Autodesk Inventor part; units mm, degrees
(part 2 of 2)
sketch "Sketch11" plane through (0, 0, 0) normal (0, -1, 0) x (1, 0, 0)
  line L0 (-38.5, 57.5) -> (38.5, 57.5) construction
  line L1 (-38.5, 57.5) -> (-38.5, -57.5) construction
  line L2 (-32.0325, -46.9289) -> (-28.4969, -50.4645)
  line L3 (-28.4969, -50.4645) -> (-32.0325, -54)
  line L4 (-32.0325, -54) -> (-35.568, -50.4645)
  line L5 (-35.568, -50.4645) -> (-32.0325, -46.9289)
  line L6 (31.4645, 54) -> (35, 54) construction
  line L7 (-38.5, -54) -> (35, -54) construction
  line L8 (35, 54) -> (-38.5, 54)
  line L9 (-38.5, 54) -> (-38.5, -54) construction
  line L10 (-22.9615, -46.9289) -> (-19.4259, -50.4645)
  line L11 (-26.497, -50.4645) -> (-22.9615, -46.9289)
  line L12 (-19.4259, -50.4645) -> (-22.9615, -54)
  line L13 (-22.9615, -54) -> (-26.497, -50.4645)
  line L14 (-13.8905, -46.9289) -> (-10.3549, -50.4645)
  line L15 (-17.426, -50.4645) -> (-13.8905, -46.9289)
  line L16 (-10.3549, -50.4645) -> (-13.8905, -54)
  line L17 (-13.8905, -54) -> (-17.426, -50.4645)
  line L18 (-4.8195, -46.9289) -> (-1.2839, -50.4645)
  line L19 (-8.355, -50.4645) -> (-4.8195, -46.9289)
  line L20 (-1.2839, -50.4645) -> (-4.8195, -54)
  line L21 (-4.8195, -54) -> (-8.355, -50.4645)
  line L22 (4.2515, -46.9289) -> (7.7871, -50.4645)
  line L23 (0.716, -50.4645) -> (4.2515, -46.9289)
  line L24 (7.7871, -50.4645) -> (4.2515, -54)
  line L25 (4.2515, -54) -> (0.716, -50.4645)
  line L26 (13.3225, -46.9289) -> (16.8581, -50.4645)
  line L27 (9.787, -50.4645) -> (13.3225, -46.9289)
  line L28 (16.8581, -50.4645) -> (13.3225, -54)
  line L29 (13.3225, -54) -> (9.787, -50.4645)
  line L30 (22.3935, -46.9289) -> (25.9291, -50.4645)
  line L31 (18.858, -50.4645) -> (22.3935, -46.9289)
  line L32 (25.9291, -50.4645) -> (22.3935, -54)
  line L33 (22.3935, -54) -> (18.858, -50.4645)
  line L34 (31.4645, -46.9289) -> (35.0001, -50.4645)
  line L35 (27.929, -50.4645) -> (31.4645, -46.9289)
  line L36 (35.0001, -50.4645) -> (31.4645, -54)
  line L37 (31.4645, -54) -> (27.929, -50.4645)
  line L38 (-32.0325, -37.9489) -> (-28.4969, -41.4845)
  line L39 (-35.568, -41.4845) -> (-32.0325, -37.9489)
  line L40 (-28.4969, -41.4845) -> (-32.0325, -45.02)
  line L41 (-32.0325, -45.02) -> (-35.568, -41.4845)
  line L42 (-22.9615, -37.9489) -> (-19.4259, -41.4845)
  line L43 (-26.497, -41.4845) -> (-22.9615, -37.9489)
  line L44 (-19.4259, -41.4845) -> (-22.9615, -45.02)
  line L45 (-22.9615, -45.02) -> (-26.497, -41.4845)
  line L46 (-13.8905, -37.9489) -> (-10.3549, -41.4845)
  line L47 (-17.426, -41.4845) -> (-13.8905, -37.9489)
  line L48 (-10.3549, -41.4845) -> (-13.8905, -45.02)
  line L49 (-13.8905, -45.02) -> (-17.426, -41.4845)
  line L50 (-4.8195, -37.9489) -> (-1.2839, -41.4845)
  line L51 (-8.355, -41.4845) -> (-4.8195, -37.9489)
  line L52 (-1.2839, -41.4845) -> (-4.8195, -45.02)
  line L53 (-4.8195, -45.02) -> (-8.355, -41.4845)
  line L54 (4.2515, -37.9489) -> (7.7871, -41.4845)
  line L55 (0.716, -41.4845) -> (4.2515, -37.9489)
  line L56 (7.7871, -41.4845) -> (4.2515, -45.02)
  line L57 (4.2515, -45.02) -> (0.716, -41.4845)
  line L58 (13.3225, -37.9489) -> (16.8581, -41.4845)
  line L59 (9.787, -41.4845) -> (13.3225, -37.9489)
  line L60 (16.8581, -41.4845) -> (13.3225, -45.02)
  line L61 (13.3225, -45.02) -> (9.787, -41.4845)
  line L62 (22.3935, -37.9489) -> (25.9291, -41.4845)
  line L63 (18.858, -41.4845) -> (22.3935, -37.9489)
  line L64 (25.9291, -41.4845) -> (22.3935, -45.02)
  line L65 (22.3935, -45.02) -> (18.858, -41.4845)
  line L66 (31.4645, -37.9489) -> (35.0001, -41.4845)
  line L67 (27.929, -41.4845) -> (31.4645, -37.9489)
  line L68 (35.0001, -41.4845) -> (31.4645, -45.02)
  line L69 (31.4645, -45.02) -> (27.929, -41.4845)
  line L70 (-32.0325, -28.9689) -> (-28.4969, -32.5045)
  line L71 (-35.568, -32.5045) -> (-32.0325, -28.9689)
  line L72 (-28.4969, -32.5045) -> (-32.0325, -36.04)
  line L73 (-32.0325, -36.04) -> (-35.568, -32.5045)
  line L74 (-22.9615, -28.9689) -> (-19.4259, -32.5045)
  line L75 (-26.497, -32.5045) -> (-22.9615, -28.9689)
  line L76 (-19.4259, -32.5045) -> (-22.9615, -36.04)
  line L77 (-22.9615, -36.04) -> (-26.497, -32.5045)
  line L78 (-13.8905, -28.9689) -> (-10.3549, -32.5045)
  line L79 (-17.426, -32.5045) -> (-13.8905, -28.9689)
  line L80 (-10.3549, -32.5045) -> (-13.8905, -36.04)
  line L81 (-13.8905, -36.04) -> (-17.426, -32.5045)
  line L82 (-4.8195, -28.9689) -> (-1.2839, -32.5045)
  line L83 (-8.355, -32.5045) -> (-4.8195, -28.9689)
  line L84 (-1.2839, -32.5045) -> (-4.8195, -36.04)
  line L85 (-4.8195, -36.04) -> (-8.355, -32.5045)
  line L86 (4.2515, -28.9689) -> (7.7871, -32.5045)
  line L87 (0.716, -32.5045) -> (4.2515, -28.9689)
  line L88 (7.7871, -32.5045) -> (4.2515, -36.04)
  line L89 (4.2515, -36.04) -> (0.716, -32.5045)
  line L90 (13.3225, -28.9689) -> (16.8581, -32.5045)
  line L91 (9.787, -32.5045) -> (13.3225, -28.9689)
  line L92 (16.8581, -32.5045) -> (13.3225, -36.04)
  line L93 (13.3225, -36.04) -> (9.787, -32.5045)
  line L94 (22.3935, -28.9689) -> (25.9291, -32.5045)
  line L95 (18.858, -32.5045) -> (22.3935, -28.9689)
  line L96 (25.9291, -32.5045) -> (22.3935, -36.04)
  line L97 (22.3935, -36.04) -> (18.858, -32.5045)
  line L98 (31.4645, -28.9689) -> (35.0001, -32.5045)
  line L99 (27.929, -32.5045) -> (31.4645, -28.9689)
  line L100 (35.0001, -32.5045) -> (31.4645, -36.04)
  line L101 (31.4645, -36.04) -> (27.929, -32.5045)
  line L102 (-32.0325, -19.9889) -> (-28.4969, -23.5245)
  line L103 (-35.568, -23.5245) -> (-32.0325, -19.9889)
  line L104 (-28.4969, -23.5245) -> (-32.0325, -27.06)
  line L105 (-32.0325, -27.06) -> (-35.568, -23.5245)
  line L106 (-22.9615, -19.9889) -> (-19.4259, -23.5245)
  line L107 (-26.497, -23.5245) -> (-22.9615, -19.9889)
  line L108 (-19.4259, -23.5245) -> (-22.9615, -27.06)
  line L109 (-22.9615, -27.06) -> (-26.497, -23.5245)
  line L110 (-13.8905, -19.9889) -> (-10.3549, -23.5245)
  line L111 (-17.426, -23.5245) -> (-13.8905, -19.9889)
  line L112 (-10.3549, -23.5245) -> (-13.8905, -27.06)
  line L113 (-13.8905, -27.06) -> (-17.426, -23.5245)
  line L114 (-4.8195, -19.9889) -> (-1.2839, -23.5245)
  line L115 (-8.355, -23.5245) -> (-4.8195, -19.9889)
  line L116 (-1.2839, -23.5245) -> (-4.8195, -27.06)
  line L117 (-4.8195, -27.06) -> (-8.355, -23.5245)
  line L118 (4.2515, -19.9889) -> (7.7871, -23.5245)
  line L119 (0.716, -23.5245) -> (4.2515, -19.9889)
  line L120 (7.7871, -23.5245) -> (4.2515, -27.06)
  line L121 (4.2515, -27.06) -> (0.716, -23.5245)
  line L122 (13.3225, -19.9889) -> (16.8581, -23.5245)
  line L123 (9.787, -23.5245) -> (13.3225, -19.9889)
  line L124 (16.8581, -23.5245) -> (13.3225, -27.06)
  line L125 (13.3225, -27.06) -> (9.787, -23.5245)
  line L126 (22.3935, -19.9889) -> (25.9291, -23.5245)
  line L127 (18.858, -23.5245) -> (22.3935, -19.9889)
  line L128 (25.9291, -23.5245) -> (22.3935, -27.06)
  line L129 (22.3935, -27.06) -> (18.858, -23.5245)
  line L130 (31.4645, -19.9889) -> (35.0001, -23.5245)
  line L131 (27.929, -23.5245) -> (31.4645, -19.9889)
  line L132 (35.0001, -23.5245) -> (31.4645, -27.06)
  line L133 (31.4645, -27.06) -> (27.929, -23.5245)
  line L134 (-32.0325, -11.0089) -> (-28.4969, -14.5445)
  line L135 (-35.568, -14.5445) -> (-32.0325, -11.0089)
  line L136 (-28.4969, -14.5445) -> (-32.0325, -18.08)
  line L137 (-32.0325, -18.08) -> (-35.568, -14.5445)
  line L138 (-22.9615, -11.0089) -> (-19.4259, -14.5445)
  line L139 (-26.497, -14.5445) -> (-22.9615, -11.0089)
  line L140 (-19.4259, -14.5445) -> (-22.9615, -18.08)
  line L141 (-22.9615, -18.08) -> (-26.497, -14.5445)
  line L142 (-13.8905, -11.0089) -> (-10.3549, -14.5445)
  line L143 (-17.426, -14.5445) -> (-13.8905, -11.0089)
  line L144 (-10.3549, -14.5445) -> (-13.8905, -18.08)
  line L145 (-13.8905, -18.08) -> (-17.426, -14.5445)
  line L146 (-4.8195, -11.0089) -> (-1.2839, -14.5445)
  line L147 (-8.355, -14.5445) -> (-4.8195, -11.0089)
  line L148 (-1.2839, -14.5445) -> (-4.8195, -18.08)
  line L149 (-4.8195, -18.08) -> (-8.355, -14.5445)
  line L150 (4.2515, -11.0089) -> (7.7871, -14.5445)
  line L151 (0.716, -14.5445) -> (4.2515, -11.0089)
  line L152 (7.7871, -14.5445) -> (4.2515, -18.08)
  line L153 (4.2515, -18.08) -> (0.716, -14.5445)
  line L154 (13.3225, -11.0089) -> (16.8581, -14.5445)
  line L155 (9.787, -14.5445) -> (13.3225, -11.0089)
  line L156 (16.8581, -14.5445) -> (13.3225, -18.08)
  line L157 (13.3225, -18.08) -> (9.787, -14.5445)
  line L158 (22.3935, -11.0089) -> (25.9291, -14.5445)
  line L159 (18.858, -14.5445) -> (22.3935, -11.0089)
  line L160 (25.9291, -14.5445) -> (22.3935, -18.08)
  line L161 (22.3935, -18.08) -> (18.858, -14.5445)
  line L162 (31.4645, -11.0089) -> (35.0001, -14.5445)
  line L163 (27.929, -14.5445) -> (31.4645, -11.0089)
  line L164 (35.0001, -14.5445) -> (31.4645, -18.08)
  line L165 (31.4645, -18.08) -> (27.929, -14.5445)
  line L166 (-38.5, -57.5) -> (-38.5, 57.5) construction
  line L167 (-38.5, 0) -> (38.5, 0) construction
  line L168 (-31.0325, -45.9745) -> (-27.497, -49.51)
  line L169 (-27.497, -49.51) -> (-23.9614, -45.9745)
  line L170 (-23.9614, -45.9745) -> (-27.497, -42.4389)
  line L171 (-27.497, -42.4389) -> (-31.0325, -45.9745)
  line L172 (-18.426, -49.51) -> (-14.8904, -45.9745)
  line L173 (-14.8904, -45.9745) -> (-18.426, -42.4389)
  line L174 (-21.9615, -45.9745) -> (-18.426, -49.51)
  line L175 (-18.426, -42.4389) -> (-21.9615, -45.9745)
  line L176 (-9.355, -49.51) -> (-5.8194, -45.9745)
  line L177 (-5.8194, -45.9745) -> (-9.355, -42.4389)
  line L178 (-12.8905, -45.9745) -> (-9.355, -49.51)
  line L179 (-9.355, -42.4389) -> (-12.8905, -45.9745)
  line L180 (-0.284, -49.51) -> (3.2516, -45.9745)
  line L181 (3.2516, -45.9745) -> (-0.284, -42.4389)
  line L182 (-3.8195, -45.9745) -> (-0.284, -49.51)
  line L183 (-0.284, -42.4389) -> (-3.8195, -45.9745)
  line L184 (8.787, -49.51) -> (12.3226, -45.9745)
  line L185 (12.3226, -45.9745) -> (8.787, -42.4389)
  line L186 (5.2515, -45.9745) -> (8.787, -49.51)
  line L187 (8.787, -42.4389) -> (5.2515, -45.9745)
  line L188 (17.858, -49.51) -> (21.3936, -45.9745)
  line L189 (21.3936, -45.9745) -> (17.858, -42.4389)
  line L190 (14.3225, -45.9745) -> (17.858, -49.51)
  line L191 (17.858, -42.4389) -> (14.3225, -45.9745)
  line L192 (26.929, -49.51) -> (30.4646, -45.9745)
  line L193 (30.4646, -45.9745) -> (26.929, -42.4389)
  line L194 (23.3935, -45.9745) -> (26.929, -49.51)
  line L195 (26.929, -42.4389) -> (23.3935, -45.9745)
  line L196 (-27.497, -40.53) -> (-23.9614, -36.9945)
  line L197 (-23.9614, -36.9945) -> (-27.497, -33.4589)
  line L198 (-31.0325, -36.9945) -> (-27.497, -40.53)
  line L199 (-27.497, -33.4589) -> (-31.0325, -36.9945)
  line L200 (-18.426, -40.53) -> (-14.8904, -36.9945)
  line L201 (-14.8904, -36.9945) -> (-18.426, -33.4589)
  line L202 (-21.9615, -36.9945) -> (-18.426, -40.53)
  line L203 (-18.426, -33.4589) -> (-21.9615, -36.9945)
  line L204 (-9.355, -40.53) -> (-5.8194, -36.9945)
  line L205 (-5.8194, -36.9945) -> (-9.355, -33.4589)
  line L206 (-12.8905, -36.9945) -> (-9.355, -40.53)
  line L207 (-9.355, -33.4589) -> (-12.8905, -36.9945)
  line L208 (-0.284, -40.53) -> (3.2516, -36.9945)
  line L209 (3.2516, -36.9945) -> (-0.284, -33.4589)
  line L210 (-3.8195, -36.9945) -> (-0.284, -40.53)
  line L211 (-0.284, -33.4589) -> (-3.8195, -36.9945)
  line L212 (8.787, -40.53) -> (12.3226, -36.9945)
  line L213 (12.3226, -36.9945) -> (8.787, -33.4589)
  line L214 (5.2515, -36.9945) -> (8.787, -40.53)
  line L215 (8.787, -33.4589) -> (5.2515, -36.9945)
  line L216 (17.858, -40.53) -> (21.3936, -36.9945)
  line L217 (21.3936, -36.9945) -> (17.858, -33.4589)
  line L218 (14.3225, -36.9945) -> (17.858, -40.53)
  line L219 (17.858, -33.4589) -> (14.3225, -36.9945)
  line L220 (26.929, -40.53) -> (30.4646, -36.9945)
  line L221 (30.4646, -36.9945) -> (26.929, -33.4589)
  line L222 (23.3935, -36.9945) -> (26.929, -40.53)
  line L223 (26.929, -33.4589) -> (23.3935, -36.9945)
  line L224 (-27.497, -31.55) -> (-23.9614, -28.0145)
  line L225 (-23.9614, -28.0145) -> (-27.497, -24.4789)
  line L226 (-31.0325, -28.0145) -> (-27.497, -31.55)
  line L227 (-27.497, -24.4789) -> (-31.0325, -28.0145)
  line L228 (-18.426, -31.55) -> (-14.8904, -28.0145)
  line L229 (-14.8904, -28.0145) -> (-18.426, -24.4789)
  line L230 (-21.9615, -28.0145) -> (-18.426, -31.55)
  line L231 (-18.426, -24.4789) -> (-21.9615, -28.0145)
  line L232 (-9.355, -31.55) -> (-5.8194, -28.0145)
  line L233 (-5.8194, -28.0145) -> (-9.355, -24.4789)
  line L234 (-12.8905, -28.0145) -> (-9.355, -31.55)
  line L235 (-9.355, -24.4789) -> (-12.8905, -28.0145)
  line L236 (-0.284, -31.55) -> (3.2516, -28.0145)
  line L237 (3.2516, -28.0145) -> (-0.284, -24.4789)
  line L238 (-3.8195, -28.0145) -> (-0.284, -31.55)
  line L239 (-0.284, -24.4789) -> (-3.8195, -28.0145)
  line L240 (8.787, -31.55) -> (12.3226, -28.0145)
  line L241 (12.3226, -28.0145) -> (8.787, -24.4789)
  line L242 (5.2515, -28.0145) -> (8.787, -31.55)
  line L243 (8.787, -24.4789) -> (5.2515, -28.0145)
  line L244 (17.858, -31.55) -> (21.3936, -28.0145)
  line L245 (21.3936, -28.0145) -> (17.858, -24.4789)
  line L246 (14.3225, -28.0145) -> (17.858, -31.55)
  line L247 (17.858, -24.4789) -> (14.3225, -28.0145)
  line L248 (26.929, -31.55) -> (30.4646, -28.0145)
  line L249 (30.4646, -28.0145) -> (26.929, -24.4789)
  line L250 (23.3935, -28.0145) -> (26.929, -31.55)
  line L251 (26.929, -24.4789) -> (23.3935, -28.0145)
  line L252 (-27.497, -22.57) -> (-23.9614, -19.0345)
  line L253 (-23.9614, -19.0345) -> (-27.497, -15.4989)
  line L254 (-31.0325, -19.0345) -> (-27.497, -22.57)
  line L255 (-27.497, -15.4989) -> (-31.0325, -19.0345)
  line L256 (-18.426, -22.57) -> (-14.8904, -19.0345)
  line L257 (-14.8904, -19.0345) -> (-18.426, -15.4989)
  line L258 (-21.9615, -19.0345) -> (-18.426, -22.57)
  line L259 (-18.426, -15.4989) -> (-21.9615, -19.0345)
  line L260 (-9.355, -22.57) -> (-5.8194, -19.0345)
  line L261 (-5.8194, -19.0345) -> (-9.355, -15.4989)
  line L262 (-12.8905, -19.0345) -> (-9.355, -22.57)
  line L263 (-9.355, -15.4989) -> (-12.8905, -19.0345)
  line L264 (-0.284, -22.57) -> (3.2516, -19.0345)
  line L265 (3.2516, -19.0345) -> (-0.284, -15.4989)
  line L266 (-3.8195, -19.0345) -> (-0.284, -22.57)
  line L267 (-0.284, -15.4989) -> (-3.8195, -19.0345)
  line L268 (8.787, -22.57) -> (12.3226, -19.0345)
  line L269 (12.3226, -19.0345) -> (8.787, -15.4989)
  line L270 (5.2515, -19.0345) -> (8.787, -22.57)
  line L271 (8.787, -15.4989) -> (5.2515, -19.0345)
  line L272 (17.858, -22.57) -> (21.3936, -19.0345)
  line L273 (21.3936, -19.0345) -> (17.858, -15.4989)
  line L274 (14.3225, -19.0345) -> (17.858, -22.57)
  line L275 (17.858, -15.4989) -> (14.3225, -19.0345)
  line L276 (26.929, -22.57) -> (30.4646, -19.0345)
  line L277 (30.4646, -19.0345) -> (26.929, -15.4989)
  line L278 (23.3935, -19.0345) -> (26.929, -22.57)
  line L279 (26.929, -15.4989) -> (23.3935, -19.0345)
  line L280 (-32.0325, 46.9289) -> (-28.4969, 50.4645)
  line L281 (-28.4969, 50.4645) -> (-32.0325, 54)
  line L282 (-32.0325, 54) -> (-35.568, 50.4645)
  line L283 (-35.568, 50.4645) -> (-32.0325, 46.9289)
  line L284 (-38.5, 54) -> (-32.0325, 54) construction
  line L285 (-38.5, 54) -> (35, 54) construction
  line L286 (-22.9615, 46.9289) -> (-19.4259, 50.4645)
  line L287 (-26.497, 50.4645) -> (-22.9615, 46.9289)
  line L288 (-19.4259, 50.4645) -> (-22.9615, 54)
  line L289 (-22.9615, 54) -> (-26.497, 50.4645)
  line L290 (-13.8905, 46.9289) -> (-10.3549, 50.4645)
  line L291 (-17.426, 50.4645) -> (-13.8905, 46.9289)
  line L292 (-10.3549, 50.4645) -> (-13.8905, 54)
  line L293 (-13.8905, 54) -> (-17.426, 50.4645)
  line L294 (-4.8195, 46.9289) -> (-1.2839, 50.4645)
  line L295 (-8.355, 50.4645) -> (-4.8195, 46.9289)
  line L296 (-1.2839, 50.4645) -> (-4.8195, 54)
  line L297 (-4.8195, 54) -> (-8.355, 50.4645)
  line L298 (4.2515, 46.9289) -> (7.7871, 50.4645)
  line L299 (0.716, 50.4645) -> (4.2515, 46.9289)
  line L300 (7.7871, 50.4645) -> (4.2515, 54)
  line L301 (4.2515, 54) -> (0.716, 50.4645)
  line L302 (13.3225, 46.9289) -> (16.8581, 50.4645)
  line L303 (9.787, 50.4645) -> (13.3225, 46.9289)
  line L304 (16.8581, 50.4645) -> (13.3225, 54)
  line L305 (13.3225, 54) -> (9.787, 50.4645)
  line L306 (22.3935, 46.9289) -> (25.9291, 50.4645)
  line L307 (18.858, 50.4645) -> (22.3935, 46.9289)
  line L308 (25.9291, 50.4645) -> (22.3935, 54)
  line L309 (22.3935, 54) -> (18.858, 50.4645)
  line L310 (31.4645, 46.9289) -> (35.0001, 50.4645)
  line L311 (27.929, 50.4645) -> (31.4645, 46.9289)
  line L312 (35.0001, 50.4645) -> (31.4645, 54)
  line L313 (31.4645, 54) -> (27.929, 50.4645)
  line L314 (-32.0325, 37.9489) -> (-28.4969, 41.4845)
  line L315 (-35.568, 41.4845) -> (-32.0325, 37.9489)
  line L316 (-28.4969, 41.4845) -> (-32.0325, 45.02)
  line L317 (-32.0325, 45.02) -> (-35.568, 41.4845)
  line L318 (-22.9615, 37.9489) -> (-19.4259, 41.4845)
  line L319 (-26.497, 41.4845) -> (-22.9615, 37.9489)
  line L320 (-19.4259, 41.4845) -> (-22.9615, 45.02)
  line L321 (-22.9615, 45.02) -> (-26.497, 41.4845)
  line L322 (-13.8905, 37.9489) -> (-10.3549, 41.4845)
  line L323 (-17.426, 41.4845) -> (-13.8905, 37.9489)
  line L324 (-10.3549, 41.4845) -> (-13.8905, 45.02)
  line L325 (-13.8905, 45.02) -> (-17.426, 41.4845)
  line L326 (-4.8195, 37.9489) -> (-1.2839, 41.4845)
  line L327 (-8.355, 41.4845) -> (-4.8195, 37.9489)
  line L328 (-1.2839, 41.4845) -> (-4.8195, 45.02)
  line L329 (-4.8195, 45.02) -> (-8.355, 41.4845)
  line L330 (4.2515, 37.9489) -> (7.7871, 41.4845)
  line L331 (0.716, 41.4845) -> (4.2515, 37.9489)
  line L332 (7.7871, 41.4845) -> (4.2515, 45.02)
  line L333 (4.2515, 45.02) -> (0.716, 41.4845)
  line L334 (13.3225, 37.9489) -> (16.8581, 41.4845)
  line L335 (9.787, 41.4845) -> (13.3225, 37.9489)
  line L336 (16.8581, 41.4845) -> (13.3225, 45.02)
  line L337 (13.3225, 45.02) -> (9.787, 41.4845)
  line L338 (22.3935, 37.9489) -> (25.9291, 41.4845)
  line L339 (18.858, 41.4845) -> (22.3935, 37.9489)
  line L340 (25.9291, 41.4845) -> (22.3935, 45.02)
  line L341 (22.3935, 45.02) -> (18.858, 41.4845)
  line L342 (31.4645, 37.9489) -> (35.0001, 41.4845)
  line L343 (27.929, 41.4845) -> (31.4645, 37.9489)
  line L344 (35.0001, 41.4845) -> (31.4645, 45.02)
  line L345 (31.4645, 45.02) -> (27.929, 41.4845)
  line L346 (-32.0325, 28.9689) -> (-28.4969, 32.5045)
  line L347 (-35.568, 32.5045) -> (-32.0325, 28.9689)
  line L348 (-28.4969, 32.5045) -> (-32.0325, 36.04)
  line L349 (-32.0325, 36.04) -> (-35.568, 32.5045)
  line L350 (-22.9615, 28.9689) -> (-19.4259, 32.5045)
  line L351 (-26.497, 32.5045) -> (-22.9615, 28.9689)
  line L352 (-19.4259, 32.5045) -> (-22.9615, 36.04)
  line L353 (-22.9615, 36.04) -> (-26.497, 32.5045)
  line L354 (-13.8905, 28.9689) -> (-10.3549, 32.5045)
  line L355 (-17.426, 32.5045) -> (-13.8905, 28.9689)
  line L356 (-10.3549, 32.5045) -> (-13.8905, 36.04)
  line L357 (-13.8905, 36.04) -> (-17.426, 32.5045)
  line L358 (-4.8195, 28.9689) -> (-1.2839, 32.5045)
  line L359 (-8.355, 32.5045) -> (-4.8195, 28.9689)
  line L360 (-1.2839, 32.5045) -> (-4.8195, 36.04)
  line L361 (-4.8195, 36.04) -> (-8.355, 32.5045)
  line L362 (4.2515, 28.9689) -> (7.7871, 32.5045)
  line L363 (0.716, 32.5045) -> (4.2515, 28.9689)
  line L364 (7.7871, 32.5045) -> (4.2515, 36.04)
  line L365 (4.2515, 36.04) -> (0.716, 32.5045)
  line L366 (13.3225, 28.9689) -> (16.8581, 32.5045)
  line L367 (9.787, 32.5045) -> (13.3225, 28.9689)
  line L368 (16.8581, 32.5045) -> (13.3225, 36.04)
  line L369 (13.3225, 36.04) -> (9.787, 32.5045)
  line L370 (22.3935, 28.9689) -> (25.9291, 32.5045)
  line L371 (18.858, 32.5045) -> (22.3935, 28.9689)
  line L372 (25.9291, 32.5045) -> (22.3935, 36.04)
  line L373 (22.3935, 36.04) -> (18.858, 32.5045)
  line L374 (31.4645, 28.9689) -> (35.0001, 32.5045)
  line L375 (27.929, 32.5045) -> (31.4645, 28.9689)
  line L376 (35.0001, 32.5045) -> (31.4645, 36.04)
  line L377 (31.4645, 36.04) -> (27.929, 32.5045)
  line L378 (-32.0325, 19.9889) -> (-28.4969, 23.5245)
  line L379 (-35.568, 23.5245) -> (-32.0325, 19.9889)
  line L380 (-28.4969, 23.5245) -> (-32.0325, 27.06)
  line L381 (-32.0325, 27.06) -> (-35.568, 23.5245)
  line L382 (-22.9615, 19.9889) -> (-19.4259, 23.5245)
  line L383 (-26.497, 23.5245) -> (-22.9615, 19.9889)
  line L384 (-19.4259, 23.5245) -> (-22.9615, 27.06)
  line L385 (-22.9615, 27.06) -> (-26.497, 23.5245)
  line L386 (-13.8905, 19.9889) -> (-10.3549, 23.5245)
  line L387 (-17.426, 23.5245) -> (-13.8905, 19.9889)
  line L388 (-10.3549, 23.5245) -> (-13.8905, 27.06)
  line L389 (-13.8905, 27.06) -> (-17.426, 23.5245)
  line L390 (-4.8195, 19.9889) -> (-1.2839, 23.5245)
  line L391 (-8.355, 23.5245) -> (-4.8195, 19.9889)
  line L392 (-1.2839, 23.5245) -> (-4.8195, 27.06)
  line L393 (-4.8195, 27.06) -> (-8.355, 23.5245)
  line L394 (4.2515, 19.9889) -> (7.7871, 23.5245)
  line L395 (0.716, 23.5245) -> (4.2515, 19.9889)
  line L396 (7.7871, 23.5245) -> (4.2515, 27.06)
  line L397 (4.2515, 27.06) -> (0.716, 23.5245)
  line L398 (13.3225, 19.9889) -> (16.8581, 23.5245)
  line L399 (9.787, 23.5245) -> (13.3225, 19.9889)
  line L400 (16.8581, 23.5245) -> (13.3225, 27.06)
  line L401 (13.3225, 27.06) -> (9.787, 23.5245)
  line L402 (22.3935, 19.9889) -> (25.9291, 23.5245)
  line L403 (18.858, 23.5245) -> (22.3935, 19.9889)
  line L404 (25.9291, 23.5245) -> (22.3935, 27.06)
  line L405 (22.3935, 27.06) -> (18.858, 23.5245)
  line L406 (31.4645, 19.9889) -> (35.0001, 23.5245)
  line L407 (27.929, 23.5245) -> (31.4645, 19.9889)
  line L408 (35.0001, 23.5245) -> (31.4645, 27.06)
  line L409 (31.4645, 27.06) -> (27.929, 23.5245)
  line L410 (-32.0325, 11.0089) -> (-28.4969, 14.5445)
  line L411 (-35.568, 14.5445) -> (-32.0325, 11.0089)
  line L412 (-28.4969, 14.5445) -> (-32.0325, 18.08)
  line L413 (-32.0325, 18.08) -> (-35.568, 14.5445)
  line L414 (-22.9615, 11.0089) -> (-19.4259, 14.5445)
  line L415 (-26.497, 14.5445) -> (-22.9615, 11.0089)
  line L416 (-19.4259, 14.5445) -> (-22.9615, 18.08)
  line L417 (-22.9615, 18.08) -> (-26.497, 14.5445)
  line L418 (-13.8905, 11.0089) -> (-10.3549, 14.5445)
  line L419 (-17.426, 14.5445) -> (-13.8905, 11.0089)
  line L420 (-10.3549, 14.5445) -> (-13.8905, 18.08)
  line L421 (-13.8905, 18.08) -> (-17.426, 14.5445)
  line L422 (-4.8195, 11.0089) -> (-1.2839, 14.5445)
  line L423 (-8.355, 14.5445) -> (-4.8195, 11.0089)
  line L424 (-1.2839, 14.5445) -> (-4.8195, 18.08)
  line L425 (-4.8195, 18.08) -> (-8.355, 14.5445)
  line L426 (4.2515, 11.0089) -> (7.7871, 14.5445)
  line L427 (0.716, 14.5445) -> (4.2515, 11.0089)
  line L428 (7.7871, 14.5445) -> (4.2515, 18.08)
  line L429 (4.2515, 18.08) -> (0.716, 14.5445)
  line L430 (13.3225, 11.0089) -> (16.8581, 14.5445)
  line L431 (9.787, 14.5445) -> (13.3225, 11.0089)
  line L432 (16.8581, 14.5445) -> (13.3225, 18.08)
  line L433 (13.3225, 18.08) -> (9.787, 14.5445)
  line L434 (22.3935, 11.0089) -> (25.9291, 14.5445)
  line L435 (18.858, 14.5445) -> (22.3935, 11.0089)
  line L436 (25.9291, 14.5445) -> (22.3935, 18.08)
  line L437 (22.3935, 18.08) -> (18.858, 14.5445)
  line L438 (31.4645, 11.0089) -> (35.0001, 14.5445)
  line L439 (27.929, 14.5445) -> (31.4645, 11.0089)
  line L440 (35.0001, 14.5445) -> (31.4645, 18.08)
  line L441 (31.4645, 18.08) -> (27.929, 14.5445)
  line L442 (-31.0325, 45.9745) -> (-27.497, 49.51)
  line L443 (-27.497, 49.51) -> (-23.9614, 45.9745)
  line L444 (-23.9614, 45.9745) -> (-27.497, 42.4389)
  line L445 (-27.497, 42.4389) -> (-31.0325, 45.9745)
  line L446 (-18.426, 49.51) -> (-14.8904, 45.9745)
  line L447 (-14.8904, 45.9745) -> (-18.426, 42.4389)
  line L448 (-21.9615, 45.9745) -> (-18.426, 49.51)
  line L449 (-18.426, 42.4389) -> (-21.9615, 45.9745)
  line L450 (-9.355, 49.51) -> (-5.8194, 45.9745)
  line L451 (-5.8194, 45.9745) -> (-9.355, 42.4389)
  line L452 (-12.8905, 45.9745) -> (-9.355, 49.51)
  line L453 (-9.355, 42.4389) -> (-12.8905, 45.9745)
  line L454 (-0.284, 49.51) -> (3.2516, 45.9745)
  line L455 (3.2516, 45.9745) -> (-0.284, 42.4389)
  line L456 (-3.8195, 45.9745) -> (-0.284, 49.51)
  line L457 (-0.284, 42.4389) -> (-3.8195, 45.9745)
  line L458 (8.787, 49.51) -> (12.3226, 45.9745)
  line L459 (12.3226, 45.9745) -> (8.787, 42.4389)
  line L460 (5.2515, 45.9745) -> (8.787, 49.51)
  line L461 (8.787, 42.4389) -> (5.2515, 45.9745)
  line L462 (17.858, 49.51) -> (21.3936, 45.9745)
  line L463 (21.3936, 45.9745) -> (17.858, 42.4389)
  line L464 (14.3225, 45.9745) -> (17.858, 49.51)
  line L465 (17.858, 42.4389) -> (14.3225, 45.9745)
  line L466 (26.929, 49.51) -> (30.4646, 45.9745)
  line L467 (30.4646, 45.9745) -> (26.929, 42.4389)
  line L468 (23.3935, 45.9745) -> (26.929, 49.51)
  line L469 (26.929, 42.4389) -> (23.3935, 45.9745)
  line L470 (-27.497, 40.53) -> (-23.9614, 36.9945)
  line L471 (-23.9614, 36.9945) -> (-27.497, 33.4589)
  line L472 (-31.0325, 36.9945) -> (-27.497, 40.53)
  line L473 (-27.497, 33.4589) -> (-31.0325, 36.9945)
  line L474 (-18.426, 40.53) -> (-14.8904, 36.9945)
  line L475 (-14.8904, 36.9945) -> (-18.426, 33.4589)
  line L476 (-21.9615, 36.9945) -> (-18.426, 40.53)
  line L477 (-18.426, 33.4589) -> (-21.9615, 36.9945)
  line L478 (-9.355, 40.53) -> (-5.8194, 36.9945)
  line L479 (-5.8194, 36.9945) -> (-9.355, 33.4589)
  line L480 (-12.8905, 36.9945) -> (-9.355, 40.53)
  line L481 (-9.355, 33.4589) -> (-12.8905, 36.9945)
  line L482 (-0.284, 40.53) -> (3.2516, 36.9945)
  line L483 (3.2516, 36.9945) -> (-0.284, 33.4589)
  line L484 (-3.8195, 36.9945) -> (-0.284, 40.53)
  line L485 (-0.284, 33.4589) -> (-3.8195, 36.9945)
  line L486 (8.787, 40.53) -> (12.3226, 36.9945)
  line L487 (12.3226, 36.9945) -> (8.787, 33.4589)
  line L488 (5.2515, 36.9945) -> (8.787, 40.53)
  line L489 (8.787, 33.4589) -> (5.2515, 36.9945)
  line L490 (17.858, 40.53) -> (21.3936, 36.9945)
  line L491 (21.3936, 36.9945) -> (17.858, 33.4589)
  line L492 (14.3225, 36.9945) -> (17.858, 40.53)
  line L493 (17.858, 33.4589) -> (14.3225, 36.9945)
  line L494 (26.929, 40.53) -> (30.4646, 36.9945)
  line L495 (30.4646, 36.9945) -> (26.929, 33.4589)
  line L496 (23.3935, 36.9945) -> (26.929, 40.53)
  line L497 (26.929, 33.4589) -> (23.3935, 36.9945)
  line L498 (-27.497, 31.55) -> (-23.9614, 28.0145)
  line L499 (-23.9614, 28.0145) -> (-27.497, 24.4789)
  line L500 (-31.0325, 28.0145) -> (-27.497, 31.55)
  line L501 (-27.497, 24.4789) -> (-31.0325, 28.0145)
  line L502 (-18.426, 31.55) -> (-14.8904, 28.0145)
  line L503 (-14.8904, 28.0145) -> (-18.426, 24.4789)
  line L504 (-21.9615, 28.0145) -> (-18.426, 31.55)
  line L505 (-18.426, 24.4789) -> (-21.9615, 28.0145)
  line L506 (-9.355, 31.55) -> (-5.8194, 28.0145)
  line L507 (-5.8194, 28.0145) -> (-9.355, 24.4789)
  line L508 (-12.8905, 28.0145) -> (-9.355, 31.55)
  line L509 (-9.355, 24.4789) -> (-12.8905, 28.0145)
  line L510 (-0.284, 31.55) -> (3.2516, 28.0145)
  line L511 (3.2516, 28.0145) -> (-0.284, 24.4789)
  line L512 (-3.8195, 28.0145) -> (-0.284, 31.55)
  line L513 (-0.284, 24.4789) -> (-3.8195, 28.0145)
  line L514 (8.787, 31.55) -> (12.3226, 28.0145)
  line L515 (12.3226, 28.0145) -> (8.787, 24.4789)
  line L516 (5.2515, 28.0145) -> (8.787, 31.55)
  line L517 (8.787, 24.4789) -> (5.2515, 28.0145)
  line L518 (17.858, 31.55) -> (21.3936, 28.0145)
  line L519 (21.3936, 28.0145) -> (17.858, 24.4789)
  line L520 (14.3225, 28.0145) -> (17.858, 31.55)
  line L521 (17.858, 24.4789) -> (14.3225, 28.0145)
  line L522 (26.929, 31.55) -> (30.4646, 28.0145)
  line L523 (30.4646, 28.0145) -> (26.929, 24.4789)
  line L524 (23.3935, 28.0145) -> (26.929, 31.55)
  line L525 (26.929, 24.4789) -> (23.3935, 28.0145)
  line L526 (-27.497, 22.57) -> (-23.9614, 19.0345)
  line L527 (-23.9614, 19.0345) -> (-27.497, 15.4989)
  line L528 (-31.0325, 19.0345) -> (-27.497, 22.57)
  line L529 (-27.497, 15.4989) -> (-31.0325, 19.0345)
  line L530 (-18.426, 22.57) -> (-14.8904, 19.0345)
  line L531 (-14.8904, 19.0345) -> (-18.426, 15.4989)
  line L532 (-21.9615, 19.0345) -> (-18.426, 22.57)
  line L533 (-18.426, 15.4989) -> (-21.9615, 19.0345)
  line L534 (-9.355, 22.57) -> (-5.8194, 19.0345)
  line L535 (-5.8194, 19.0345) -> (-9.355, 15.4989)
  line L536 (-12.8905, 19.0345) -> (-9.355, 22.57)
  line L537 (-9.355, 15.4989) -> (-12.8905, 19.0345)
  line L538 (-0.284, 22.57) -> (3.2516, 19.0345)
  line L539 (3.2516, 19.0345) -> (-0.284, 15.4989)
  line L540 (-3.8195, 19.0345) -> (-0.284, 22.57)
  line L541 (-0.284, 15.4989) -> (-3.8195, 19.0345)
  line L542 (8.787, 22.57) -> (12.3226, 19.0345)
  line L543 (12.3226, 19.0345) -> (8.787, 15.4989)
  line L544 (5.2515, 19.0345) -> (8.787, 22.57)
  line L545 (8.787, 15.4989) -> (5.2515, 19.0345)
  line L546 (17.858, 22.57) -> (21.3936, 19.0345)
  line L547 (21.3936, 19.0345) -> (17.858, 15.4989)
  line L548 (14.3225, 19.0345) -> (17.858, 22.57)
  line L549 (17.858, 15.4989) -> (14.3225, 19.0345)
  line L550 (26.929, 22.57) -> (30.4646, 19.0345)
  line L551 (30.4646, 19.0345) -> (26.929, 15.4989)
  line L552 (23.3935, 19.0345) -> (26.929, 22.57)
  line L553 (26.929, 15.4989) -> (23.3935, 19.0345)
  line L554 (-35.568, -48.51) -> (-33.0324, -45.9745)
  line L555 (-33.0324, -45.9745) -> (-35.568, -43.4389)
  line L556 (-35.568, -43.4389) -> (-35.568, -48.51)
  line L557 (-33.0324, -36.9945) -> (-35.568, -34.4589)
  line L558 (-35.568, -34.4589) -> (-35.568, -39.53)
  line L559 (-35.568, -39.53) -> (-33.0324, -36.9945)
  line L560 (-33.0324, -28.0145) -> (-35.568, -25.4789)
  line L561 (-35.568, -25.4789) -> (-35.568, -30.55)
  line L562 (-35.568, -30.55) -> (-33.0324, -28.0145)
  line L563 (-33.0324, -19.0345) -> (-35.568, -16.4989)
  line L564 (-35.568, -16.4989) -> (-35.568, -21.57)
  line L565 (-35.568, -21.57) -> (-33.0324, -19.0345)
  line L566 (-27.497, -51.4189) -> (-24.9159, -54)
  line L567 (-30.078, -54) -> (-27.497, -51.4189)
  line L568 (-30.078, -54) -> (-24.9159, -54)
  line L569 (-21.007, -54) -> (-15.8449, -54)
  line L570 (-21.007, -54) -> (-18.426, -51.4189)
  line L571 (-18.426, -51.4189) -> (-15.8449, -54)
  line L572 (-11.936, -54) -> (-6.7739, -54)
  line L573 (-11.936, -54) -> (-9.355, -51.4189)
  line L574 (-9.355, -51.4189) -> (-6.7739, -54)
  line L575 (-2.865, -54) -> (2.2971, -54)
  line L576 (-2.865, -54) -> (-0.284, -51.4189)
  line L577 (-0.284, -51.4189) -> (2.2971, -54)
  line L578 (6.206, -54) -> (11.3681, -54)
  line L579 (6.206, -54) -> (8.787, -51.4189)
  line L580 (8.787, -51.4189) -> (11.3681, -54)
  line L581 (15.277, -54) -> (20.4391, -54)
  line L582 (15.277, -54) -> (17.858, -51.4189)
  line L583 (17.858, -51.4189) -> (20.4391, -54)
  line L584 (24.348, -54) -> (29.5101, -54)
  line L585 (24.348, -54) -> (26.929, -51.4189)
  line L586 (26.929, -51.4189) -> (29.5101, -54)
  line L587 (-35.568, -32.5045) -> (35.0001, -32.5045)
  line L588 (35, -54) -> (35, -11) construction
  line L589 (-27.497, -13.59) -> (-24.9159, -11.0089)
  line L590 (-30.078, -11.0089) -> (-27.497, -13.59)
  line L591 (-30.078, -11.0089) -> (-24.9159, -11.0089)
  line L592 (-21.007, -11.0089) -> (-15.8449, -11.0089)
  line L593 (-21.007, -11.0089) -> (-18.426, -13.59)
  line L594 (-18.426, -13.59) -> (-15.8449, -11.0089)
  line L595 (-11.936, -11.0089) -> (-6.7739, -11.0089)
  line L596 (-11.936, -11.0089) -> (-9.355, -13.59)
  line L597 (-9.355, -13.59) -> (-6.7739, -11.0089)
  line L598 (-2.865, -11.0089) -> (2.2971, -11.0089)
  line L599 (-2.865, -11.0089) -> (-0.284, -13.59)
  line L600 (-0.284, -13.59) -> (2.2971, -11.0089)
  line L601 (6.206, -11.0089) -> (11.3681, -11.0089)
  line L602 (6.206, -11.0089) -> (8.787, -13.59)
  line L603 (8.787, -13.59) -> (11.3681, -11.0089)
  line L604 (15.277, -11.0089) -> (20.4391, -11.0089)
  line L605 (15.277, -11.0089) -> (17.858, -13.59)
  line L606 (17.858, -13.59) -> (20.4391, -11.0089)
  line L607 (24.348, -11.0089) -> (29.5101, -11.0089)
  line L608 (24.348, -11.0089) -> (26.929, -13.59)
  line L609 (26.929, -13.59) -> (29.5101, -11.0089)
  line L610 (-35.568, -52.2322) -> (-33.8002, -54)
  line L611 (-35.568, -52.2322) -> (-35.568, -54)
  line L612 (-38.5, -54) -> (35, -54) construction
  line L613 (-33.8002, -54) -> (-35.568, -54)
  line L614 (-35.568, -12.7767) -> (-33.8002, -11.0089)
  line L615 (-35.568, -12.7767) -> (-35.568, -11.0089)
  line L616 (-33.8002, -11.0089) -> (-35.568, -11.0089)
  line L617 (-0.284, -69.5609) -> (-0.284, 7.1331)
  line L618 (35.0001, -48.51) -> (32.4645, -45.9745)
  line L619 (32.4645, -45.9745) -> (35.0001, -43.4389)
  line L620 (35.0001, -43.4389) -> (35.0001, -48.51)
  line L621 (32.4645, -36.9945) -> (35.0001, -34.4589)
  line L622 (35.0001, -34.4589) -> (35.0001, -39.53)
  line L623 (35.0001, -39.53) -> (32.4645, -36.9945)
  line L624 (32.4645, -28.0145) -> (35.0001, -25.4789)
  line L625 (35.0001, -25.4789) -> (35.0001, -30.55)
  line L626 (35.0001, -30.55) -> (32.4645, -28.0145)
  line L627 (32.4645, -19.0345) -> (35.0001, -16.4989)
  line L628 (35.0001, -16.4989) -> (35.0001, -21.57)
  line L629 (35.0001, -21.57) -> (32.4645, -19.0345)
  line L630 (35.0001, -52.2322) -> (33.2323, -54)
  line L631 (35.0001, -52.2322) -> (35.0001, -54)
  line L632 (33.2323, -54) -> (35.0001, -54)
  line L633 (33.2323, -11.0089) -> (35.0001, -11.0089)
  line L634 (35.0001, -12.7767) -> (33.2323, -11.0089)
  line L635 (35.0001, -12.7767) -> (35.0001, -11.0089)
  line L636 (-35.568, 48.51) -> (-33.0324, 45.9745)
  line L637 (-33.0324, 45.9745) -> (-35.568, 43.4389)
  line L638 (-35.568, 43.4389) -> (-35.568, 48.51)
  line L639 (-33.0324, 36.9945) -> (-35.568, 34.4589)
  line L640 (-35.568, 34.4589) -> (-35.568, 39.53)
  line L641 (-35.568, 39.53) -> (-33.0324, 36.9945)
  line L642 (-33.0324, 28.0145) -> (-35.568, 25.4789)
  line L643 (-35.568, 25.4789) -> (-35.568, 30.55)
  line L644 (-35.568, 30.55) -> (-33.0324, 28.0145)
  line L645 (-33.0324, 19.0345) -> (-35.568, 16.4989)
  line L646 (-35.568, 16.4989) -> (-35.568, 21.57)
  line L647 (-35.568, 21.57) -> (-33.0324, 19.0345)
  line L648 (-30.078, 54) -> (-24.9159, 54)
  line L649 (-21.007, 54) -> (-15.8449, 54)
  line L650 (-21.007, 54) -> (-18.426, 51.4189)
  line L651 (-18.426, 51.4189) -> (-15.8449, 54)
  line L652 (-11.936, 54) -> (-6.7739, 54)
  line L653 (-11.936, 54) -> (-9.355, 51.4189)
  line L654 (-9.355, 51.4189) -> (-6.7739, 54)
  line L655 (-2.865, 54) -> (2.2971, 54)
  line L656 (-2.865, 54) -> (-0.284, 51.4189)
  line L657 (-0.284, 51.4189) -> (2.2971, 54)
  line L658 (6.206, 54) -> (11.3681, 54)
  line L659 (6.206, 54) -> (8.787, 51.4189)
  line L660 (8.787, 51.4189) -> (11.3681, 54)
  line L661 (15.277, 54) -> (20.4391, 54)
  line L662 (15.277, 54) -> (17.858, 51.4189)
  line L663 (17.858, 51.4189) -> (20.4391, 54)
  line L664 (24.348, 54) -> (29.5101, 54)
  line L665 (24.348, 54) -> (26.929, 51.4189)
  line L666 (26.929, 51.4189) -> (29.5101, 54)
  line L667 (-30.078, 11.0089) -> (-24.9159, 11.0089)
  line L668 (-27.497, 13.59) -> (-24.9159, 11.0089)
  line L669 (-30.078, 11.0089) -> (-27.497, 13.59)
  line L670 (-21.007, 11.0089) -> (-15.8449, 11.0089)
  line L671 (-18.426, 13.59) -> (-15.8449, 11.0089)
  line L672 (-21.007, 11.0089) -> (-18.426, 13.59)
  line L673 (-11.936, 11.0089) -> (-6.7739, 11.0089)
  line L674 (-9.355, 13.59) -> (-6.7739, 11.0089)
  line L675 (-11.936, 11.0089) -> (-9.355, 13.59)
  line L676 (-2.865, 11.0089) -> (2.2971, 11.0089)
  line L677 (-0.284, 13.59) -> (2.2971, 11.0089)
  line L678 (-2.865, 11.0089) -> (-0.284, 13.59)
  line L679 (6.206, 11.0089) -> (11.3681, 11.0089)
  line L680 (8.787, 13.59) -> (11.3681, 11.0089)
  line L681 (6.206, 11.0089) -> (8.787, 13.59)
  line L682 (15.277, 11.0089) -> (20.4391, 11.0089)
  line L683 (17.858, 13.59) -> (20.4391, 11.0089)
  line L684 (15.277, 11.0089) -> (17.858, 13.59)
  line L685 (24.348, 11.0089) -> (26.929, 13.59)
  line L686 (26.929, 13.59) -> (29.5101, 11.0089)
  line L687 (24.348, 11.0089) -> (29.5101, 11.0089)
  line L688 (-35.568, 52.2322) -> (-33.8002, 54)
  line L689 (-35.568, 52.2322) -> (-35.568, 54)
  line L690 (-33.8002, 54) -> (-35.568, 54)
  line L691 (-33.8002, 11.0089) -> (-35.568, 11.0089)
  line L692 (-35.568, 12.7767) -> (-33.8002, 11.0089)
  line L693 (-35.568, 12.7767) -> (-35.568, 11.0089)
  line L694 (33.2323, 54) -> (35.0001, 54)
  line L695 (35.0001, 52.2322) -> (35.0001, 54)
  line L696 (35.0001, 52.2322) -> (33.2323, 54)
  line L697 (32.4645, 45.9745) -> (35.0001, 43.4389)
  line L698 (35.0001, 43.4389) -> (35.0001, 48.51)
  line L699 (35.0001, 48.51) -> (32.4645, 45.9745)
  line L700 (35.0001, 34.4589) -> (35.0001, 39.53)
  line L701 (35.0001, 39.53) -> (32.4645, 36.9945)
  line L702 (32.4645, 36.9945) -> (35.0001, 34.4589)
  line L703 (32.4645, 28.0145) -> (35.0001, 25.4789)
  line L704 (35.0001, 30.55) -> (32.4645, 28.0145)
  line L705 (35.0001, 25.4789) -> (35.0001, 30.55)
  line L706 (35.0001, 16.4989) -> (35.0001, 21.57)
  line L707 (35.0001, 21.57) -> (32.4645, 19.0345)
  line L708 (32.4645, 19.0345) -> (35.0001, 16.4989)
  line L709 (35.0001, 12.7767) -> (33.2323, 11.0089)
  line L710 (35.0001, 12.7767) -> (35.0001, 11.0089)
  line L711 (33.2323, 11.0089) -> (35.0001, 11.0089)
  line L712 (-27.497, 51.4189) -> (-24.9159, 54)
  line L713 (-30.078, 54) -> (-27.497, 51.4189)
  line L714 (-30.078, 54) -> (-24.9159, 54)
  point P0 (0, 0)
  point P1 (-32.0325, -54)
  dimension "d88" = 5
  dimension "d89" = 5
  dimension "d93" = 3.5
  dimension "d94" = 2.932
  dimension "d96" = 7.0711
  dimension "d100" = 9.071
  dimension "d103" = 8.98
  dimension "d106" = 5
  dimension "d107" = 5
  dimension "d108" = 1.382
  dimension "d109" = 1.382
  dimension "d110" = 1.382
  dimension "d111" = 1.382
  dimension "d114" = 9.071
  dimension "d117" = 8.98
  dimension "d135" = 1.382
  dimension "d155" = 1.382
  dimension "d156" = 1.382
  dimension "d159" = 8.98
  dimension "d166" = 1.382
  dimension "d167" = 1.382
  dimension "d170" = 9.071
  constraints: 1418 end point, 394 symmetric about line, 5 parallel, 5 perpendicular, 4 horizontal, 4 vertical, 1 collinear, 1 midpoint, 1 point on line, 585 other
  measures "d88" distance between parallel lines of L4 L2
  measures "d89" distance between parallel lines of L5 L3
  measures "d93" distance between parallel lines of L0 L8
  measures "d94" distance from line of L1 L4.end
  measures "d96" distance of L2.start point (-32.032, -54)
  measures "d100" distance of L2.start L10.start
  measures "d103" distance of L2.start L38.start
  measures "d106" distance between parallel lines of L171 L169
  measures "d107" distance between parallel lines of L168 L170
  measures "d108" distance between parallel lines of L2 L168
  measures "d109" distance between parallel lines of L45 L170
  measures "d110" distance between parallel lines of L40 L171
  measures "d111" distance between parallel lines of L11 L169
  measures "d114" distance of L168.end L172.start
  measures "d117" distance of L168.end L196.start
  measures "d135" distance between parallel lines of L254 L102
  measures "d155" distance between parallel lines of L554 L5
  measures "d156" distance between parallel lines of L555 L41
  measures "d159" distance of L554.end L557.start
  measures "d166" distance between parallel lines of L3 L567
  measures "d167" distance between parallel lines of L566 L13
  measures "d170" distance of L567.start L569.start
extrude "Back Swiss-ification" cut sketch "Sketch11" against normal up to surface (3.5 mm away)
body "Solid1"
